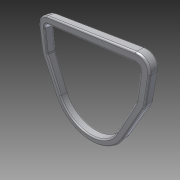
# Autodesk Inventor part: y_carryage_bearing_zip_tie
Saved by Autodesk Inventor 2014 (Build 180170000, 170)
## iProperties
Created: 2014-01-11
Part Number: y_carryage_bearing_zip_tie
Material: ABS Plastic
Document SubType Name: Modeling
Designer: buben
Density: 1.06 g/cm^3
Appearance: Smooth - White
Author: buben
Autodesk Inventor part; units mm, degrees
ref_plane "YZ Plane" through (0, 0, 0) normal (1, 0, 0) x (0, 1, 0)
ref_plane "XZ Plane" through (0, 0, 0) normal (0, 1, 0) x (-1, 0, 0)
ref_plane "XY Plane" through (0, 0, 0) normal (0, 0, 1) x (1, 0, 0)
sketch "Sketch1" plane through (0, 0, 0) normal (0, 1, 0) x (-1, 0, 0)
  line L0 (-9, 0) -> (9, 0)
  arc A0 (-9, 0) -> (-10, -1) centre (-9, -1) ccw
  line L1 (-10, -1) -> (-10, -5.6474)
  arc A1 (-10, -5.6474) -> (-9.9358, -6) centre (-9, -5.6474) ccw
  line L2 (-9.9358, -6) -> (-7.0184, -13.7433)
  arc A2 (-7.0184, -13.7433) -> (7.0184, -13.7433) centre (0, -11.099) ccw
  line L3 (7.0184, -13.7433) -> (9.9358, -6)
  arc A3 (9.9358, -6) -> (10, -5.6474) centre (9, -5.6474) ccw
  line L4 (10, -5.6474) -> (10, -1)
  arc A4 (10, -1) -> (9, 0) centre (9, -1) ccw
  line L5 (9, 1.5) -> (-9, 1.5)
  arc A5 (-9, 1.5) -> (-11.5, -1) centre (-9, -1) ccw
  line L6 (-11.5, -1) -> (-11.5, -5.6474)
  arc A6 (-11.5, -5.6474) -> (-11.3395, -6.5289) centre (-9, -5.6474) ccw
  line L7 (-11.3395, -6.5289) -> (-8.4221, -14.2721)
  arc A7 (-8.4221, -14.2721) -> (8.4221, -14.2721) centre (0, -11.099) ccw
  line L8 (8.4221, -14.2721) -> (11.3395, -6.5289)
  arc A8 (11.3395, -6.5289) -> (11.5, -5.6474) centre (9, -5.6474) ccw
  line L9 (11.5, -5.6474) -> (11.5, -1)
  arc A9 (11.5, -1) -> (9, 1.5) centre (9, -1) ccw
  point P0 (0, 0)
  point P1 (0, 0)
  dimension "d0" = 18
  dimension "d1" = 6
  dimension "d2" = 1
  dimension "d3" = 1
  dimension "d4" = 9
  dimension "d5" = 7.5
  dimension "d6" = 1
  dimension "d7" = 1
  dimension "d8" = 11.099
  dimension "d9" = 1.5
  constraints: 20 end point, 20 point on circle, 10 centre point, 10 tangent, 2 midpoint, 2 parallel, 2 perpendicular, 1 horizontal, 1 horizontal alignment, 1 vertical alignment, 9 other
  measures "d0" distance of L0.start L0.end
  measures "d1" vertical distance of L2.start L0.start
  measures "d2" radius of A0
  measures "d3" radius of A1
  measures "d4" distance of point (0, 0) L0.start
  measures "d5" radius of A2
  measures "d6" radius of A3
  measures "d7" radius of A4
  measures "d8" distance from line of L0 A2.centre
  measures "d9" distance between parallel lines of L6 L1
extrude "Extrusion1" add sketch "Sketch1" along normal blind 2
fillet "Fillet1" radius 0.3 40 edges at (10.7678, 2, 0.7678) (11.5, 2, -3.3237) (11.4595, 2, -6.0954) (9.8808, 2, -10.4005) (0, 2, -20.099) (-9.8808, 2, -10.4005) (-11.4595, 2, -6.0954) (-11.5, 2, -3.3237) (-10.7678, 2, 0.7678) (0, 2, 1.5) (10.7678, 0, 0.7678) (11.5, 0, -3.3237) (11.4595, 0, -6.0954) (9.8808, 0, -10.4005) (0, 0, -20.099) (-9.8808, 0, -10.4005) (-11.4595, 0, -6.0954) (-11.5, 0, -3.3237) (-10.7678, 0, 0.7678) (0, 0, 1.5) (-9.7071, 2, -0.2929) (-10, 2, -3.3237) (-9.9838, 2, -5.8266) (-8.4771, 2, -9.8716) (0, 2, -18.599) (8.4771, 2, -9.8716) (9.9838, 2, -5.8266) (10, 2, -3.3237) (9.7071, 2, -0.2929) (0, 2, 0) (9.7071, 0, -0.2929) (10, 0, -3.3237) (9.9838, 0, -5.8266) (8.4771, 0, -9.8716) (0, 0, -18.599) (-8.4771, 0, -9.8716) (-9.9838, 0, -5.8266) (-10, 0, -3.3237) (-9.7071, 0, -0.2929) (0, 0, 0)
equation "\"d3\" = d2"
equation "\"d4\" = 0.5 * d0"
equation "\"d6\" = d3"
equation "\"d7\" = d6"
body "Solid1"
